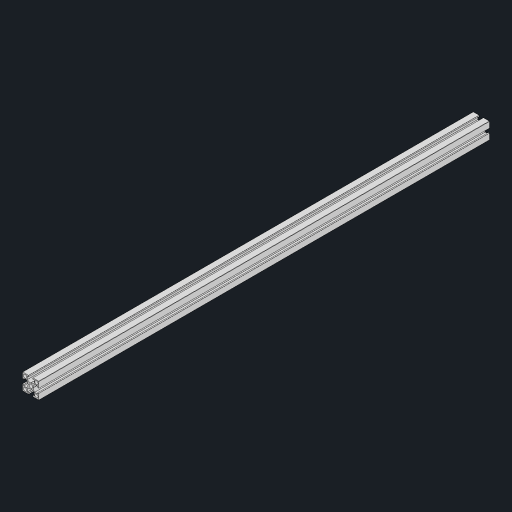
# Autodesk Inventor part: 20x20 Profile
Saved by Autodesk Inventor 2024.1 (Build 281209000, 209)
## iProperties
Created: 2024-01-10
Part Number: 20x20 Profile
Material: 일반
Document SubType Name: Modeling
Designer: KBU
Density: 1 g/cm^3
Appearance: 기본값
Author: KBU
Autodesk Inventor part; units mm, degrees
ref_plane "YZ Plane" through (0, 0, 0) normal (1, 0, 0) x (0, 1, 0)
ref_plane "XZ Plane" through (0, 0, 0) normal (0, 1, 0) x (-1, 0, 0)
ref_plane "XY Plane" through (0, 0, 0) normal (0, 0, 1) x (1, 0, 0)
sketch "스케치1" plane through (0, 0, 0) normal (0, 0, 1) x (1, 0, 0)
  line L0 (-9.7, -10) -> (9.7, -10)
  line L1 (10, -9.7) -> (10, 9.7)
  line L2 (9.7, 10) -> (-9.7, 10)
  line L3 (-10, 9.7) -> (-10, -9.7)
  line L4 (-10, -10) -> (10, 10) construction
  line L5 (10, -10) -> (-10, 10) construction
  circle A0 centre (-7, 7) radius 2
  line L6 (0, 15.6683) -> (0, -20)
  line L7 (-22.0072, 0) -> (22.0072, 0)
  circle A1 centre (0, 0) radius 2.15
  arc A2 (-9.7, 10) -> (-10, 9.7) centre (-9.7, 9.7) ccw
  arc A3 (10, 9.7) -> (9.7, 10) centre (9.7, 9.7) ccw
  arc A4 (9.7, -10) -> (10, -9.7) centre (9.7, -9.7) ccw
  arc A5 (-10, -9.7) -> (-9.7, -10) centre (-9.7, -9.7) ccw
  line L8 (-2.65, 10) -> (-2.65, 8.5)
  line L9 (-2.65, 8.5) -> (-4.15, 8.5)
  line L10 (-4.15, 8.5) -> (-4.15, 4.8)
  line L11 (4.15, 4.8) -> (4.15, 8.5)
  line L12 (4.15, 8.5) -> (2.65, 8.5)
  line L13 (2.65, 8.5) -> (2.65, 10)
  line L14 (-0.1, 3.3008) -> (0, 3.2)
  line L15 (0.1, 3.3008) -> (0, 3.2)
  arc A6 (-4.15, 4.8) -> (-0.1, 3.3008) centre (0, 9.7908) ccw
  arc A7 (0.1, 3.3008) -> (4.15, 4.8) centre (0, 9.7908) ccw
  circle A8 centre (7, 7) radius 2
  circle A9 centre (-7, -7) radius 2
  circle A10 centre (7, -7) radius 2
  line L16 (-3.3008, 0.1) -> (-3.2, 0)
  line L17 (-3.3008, -0.1) -> (-3.2, 0)
  arc A11 (-4.8, -4.15) -> (-3.3008, -0.1) centre (-9.7908, 0) ccw
  line L18 (-8.5, -4.15) -> (-4.8, -4.15)
  line L19 (-10, -2.65) -> (-8.5, -2.65)
  line L20 (-8.5, 2.65) -> (-10, 2.65)
  arc A12 (-3.3008, 0.1) -> (-4.8, 4.15) centre (-9.7908, 0) ccw
  line L21 (-4.8, 4.15) -> (-8.5, 4.15)
  line L22 (-8.5, 4.15) -> (-8.5, 2.65)
  line L23 (-8.5, -2.65) -> (-8.5, -4.15)
  line L24 (-0.1, -3.3008) -> (0, -3.2)
  line L25 (0.1, -3.3008) -> (0, -3.2)
  arc A13 (4.15, -4.8) -> (0.1, -3.3008) centre (0, -9.7908) ccw
  line L26 (4.15, -8.5) -> (4.15, -4.8)
  line L27 (2.65, -10) -> (2.65, -8.5)
  line L28 (-2.65, -8.5) -> (-2.65, -10)
  arc A14 (-0.1, -3.3008) -> (-4.15, -4.8) centre (0, -9.7908) ccw
  line L29 (-4.15, -4.8) -> (-4.15, -8.5)
  line L30 (-4.15, -8.5) -> (-2.65, -8.5)
  line L31 (2.65, -8.5) -> (4.15, -8.5)
  line L32 (3.3008, -0.1) -> (3.2, 0)
  line L33 (3.3008, 0.1) -> (3.2, 0)
  arc A15 (4.8, 4.15) -> (3.3008, 0.1) centre (9.7908, 0) ccw
  line L34 (8.5, 4.15) -> (4.8, 4.15)
  line L35 (10, 2.65) -> (8.5, 2.65)
  line L36 (8.5, -2.65) -> (10, -2.65)
  arc A16 (3.3008, -0.1) -> (4.8, -4.15) centre (9.7908, 0) ccw
  line L37 (4.8, -4.15) -> (8.5, -4.15)
  line L38 (8.5, -4.15) -> (8.5, -2.65)
  line L39 (8.5, 2.65) -> (8.5, 4.15)
  point P0 (2.65, 9.25)
  point P1 (-2.65, 9.25)
  point P2 (-4.15, 6.65)
  point P3 (0, 3.3)
  point P4 (-3.3, 0)
  point P5 (-9.25, -2.65)
  point P6 (-6.65, -4.15)
  point P7 (-9.25, 2.65)
  point P8 (0, -3.3)
  point P9 (2.65, -9.25)
  point P10 (4.15, -6.65)
  point P11 (-2.65, -9.25)
  point P12 (3.3, 0)
  point P13 (9.25, 2.65)
  point P14 (6.65, 4.15)
  point P15 (9.25, -2.65)
  dimension "d0" = 20
  dimension "d1" = 20
  dimension "d2" = 4
  dimension "d3" = 14
  dimension "d4" = 14
  dimension "d5" = 4.3
  dimension "d6" = 0.3
  dimension "d9" = 8.3
  dimension "d10" = 5.3
  dimension "d11" = 5.3
  dimension "d12" = 1.5
  dimension "d15" = 0.1
  dimension "d16" = 0.1
  dimension "d17" = 0.1
  dimension "d19" = 3.7
  dimension "d22" = 360
  constraints: 80 end point, 28 point on circle, 21 point on line, 17 centre point, 8 tangent, 6 midpoint, 4 perpendicular, 3 equal radius, 3 symmetric about line, 2 horizontal, 2 parallel, 2 vertical, 1 coincident, 108 other
  measures "d0" distance of L5.start L4.end
  measures "d1" distance of L4.end L5.end
  measures "d2" diameter of A0
  measures "d3" diameter of A0.centre L6
  measures "d4" diameter of A0.centre L7
  measures "d5" diameter of A1
  measures "d6" radius of A2
  measures "d9" diameter of point (-4.15, 6.65) L6
  measures "d10" diameter of L8 L6
  measures "d11" diameter of L13 L6
  measures "d12" distance of L8.start L8.end
  measures "d15" distance of point (0, 3.3) L14.end
  measures "d16" distance of point (0, 3.3) L14.start
  measures "d17" distance of L15.start point (0, 3.3)
  measures "d19" distance of L11.start L11.end
extrude "프로파일 길이 설정" add sketch "스케치1" along normal blind 550 contours A5 L3 L19 L23 L18 A11 L17 L7 A1 L6 L24 A14 L29 L30 L28 L0 | L27 L31 L26 A13 L25 L6 A1 L7 L32 A16 L37 L38 L36 L1 A4 L0 | L3 A2 L2 L8 L9 L10 A6 L14 L6 A1 L7 L16 A12 L21 L22 L20 | A1 L6 L15 A7 L11 L12 L13 L2 A3 L1 L35 L39 L34 A15 L33 L7
fillet "모서리" radius 0.05 32 edges at (10, 2.65, 275) (8.5, 2.65, 275) (8.5, 4.15, 275) (10, -2.65, 275) (8.5, -2.65, 275) (8.5, -4.15, 275) (2.65, 8.5, 275) (2.65, 10, 275) (4.15, 8.5, 275) (-4.15, 8.5, 275) (-2.65, 8.5, 275) (-2.65, 10, 275) (-10, 2.65, 275) (-8.5, 2.65, 275) (-8.5, 4.15, 275) (-8.5, -4.15, 275) (-8.5, -2.65, 275) (-10, -2.65, 275) (-2.65, -10, 275) (-2.65, -8.5, 275) (-4.15, -8.5, 275) (2.65, -8.5, 275) (4.15, -8.5, 275) (2.65, -10, 275) (4.15, -4.8, 275) (-4.15, -4.8, 275) (-4.8, -4.15, 275) (-4.8, 4.15, 275) (-4.15, 4.8, 275) (4.15, 4.8, 275) (4.8, -4.15, 275) (4.8, 4.15, 275)
equation "\"d0\" = d1"
equation "\"d11\" = d10"
equation "\"d17\" = d16"
